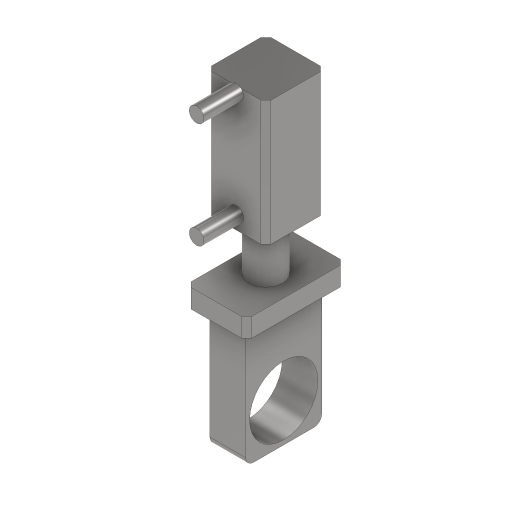
# Autodesk Inventor part: Gatevalve_70_pneumatic
Saved by Autodesk Inventor 2024.2 (Build 282272000, 272)
## iProperties
Created: 2022-11-16
Part Number: Gatevalve_70_pneumatic
Material: Stainless Steel, 440C
Document SubType Name: Modeling
Designer: kuzmin
Density: 7.75 g/cm^3
Appearance: Semi-Polished
Author: kuzmin
Autodesk Inventor part; units mm, degrees
ref_plane "YZ Plane" through (0, 0, 0) normal (1, 0, 0) x (0, 1, 0)
ref_plane "XZ Plane" through (0, 0, 0) normal (0, 1, 0) x (-1, 0, 0)
ref_plane "XY Plane" through (0, 0, 0) normal (0, 0, 1) x (1, 0, 0)
sketch "Sketch1" plane through (0, 0, 0) normal (0, 1, 0) x (-1, 0, 0)
  line L0 (18, 38.5) -> (-18, 38.5)
  line L1 (-18, 38.5) -> (-18, -38.5)
  line L2 (-18, -38.5) -> (18, -38.5)
  line L3 (18, -38.5) -> (18, 38.5)
  line L4 (18, 38.5) -> (-18, -38.5) construction
  point P0 (0, 0)
  point P1 (0, 0)
  dimension "d0" = 77
  dimension "d1" = 36
  constraints: 10 end point, 2 parallel, 1 coincident, 1 horizontal, 1 midpoint, 1 perpendicular
  measures "d0" distance of L2.end L0.start
  measures "d1" distance of L1.end L2.end
extrude "Extrusion1" add sketch "Sketch1" along normal blind 122
sketch "Sketch2" plane through (0, 122, 0) normal (0, 1, 0) x (1, 0, 0)
  line L0 (-30.5, -50) -> (30.5, -50)
  line L1 (30.5, -50) -> (30.5, 50)
  line L2 (30.5, 50) -> (-30.5, 50)
  line L3 (-30.5, 50) -> (-30.5, -50)
  line L4 (-30.5, 50) -> (30.5, -50) construction
  point P0 (0, 0)
  point P1 (0, 0)
  dimension "d4" = 100
  dimension "d5" = 61
  constraints: 10 end point, 2 parallel, 1 coincident, 1 horizontal, 1 midpoint, 1 perpendicular
  measures "d4" distance of L2.end L0.start
  measures "d5" distance of L1.end L2.end
extrude "Extrusion2" add sketch "Sketch2" along normal blind 19
sketch "Sketch3" plane through (0, 141, 0) normal (0, 1, 0) x (1, 0, 0)
  circle A0 centre (0, 0) radius 17
  dimension "d8" = 34
  constraints: 1 centre point, 1 coincident
  measures "d8" diameter of A0
extrude "Extrusion3" add sketch "Sketch3" along normal blind 53
sketch "Sketch4" plane through (0, 194, 0) normal (0, 1, 0) x (1, 0, 0)
  line L0 (-30, -30) -> (30, -30)
  line L1 (30, -30) -> (30, 30)
  line L2 (30, 30) -> (-30, 30)
  line L3 (-30, 30) -> (-30, -30)
  line L4 (-30, 30) -> (30, -30) construction
  point P0 (0, 0)
  point P1 (0, 0)
  dimension "d11" = 60
  constraints: 10 end point, 2 parallel, 2 perpendicular, 1 coincident, 1 horizontal, 1 midpoint
  measures "d11" distance of L2.end L0.start
extrude "Extrusion4" add sketch "Sketch4" along normal blind 126
sketch "Sketch5" plane through (-30, 194, 30) normal (0, 0, 1) x (1, 0, 0)
  circle A0 centre (30, 14) radius 7.5
  line L0 (0, 0) -> (60, 0) projected
  circle A1 centre (30, 121) radius 7.5
  line L1 (0, 126) -> (60, 126) projected
  point P0 (30, -194)
  point P1 (30, 0)
  point P2 (30, 126)
  point P3 (35.5902, 126)
  point P4 (24.4098, 126)
  dimension "d14" = 15
  dimension "d15" = 14
  dimension "d16" = 5
  constraints: 2 centre point, 2 midpoint, 2 vertical alignment, 1 equal radius
  measures "d14" diameter of A0
  measures "d15" distance from line of L0 A0.centre
  measures "d16" distance from line of L1 A1.centre
extrude "Extrusion5" add sketch "Sketch5" along normal blind 40
chamfer "Chamfer1" distance 5 angle 45 4 edges at (30, 257, 30) (30, 257, -30) (-30, 257, -30) (-30, 257, 30)
chamfer "Chamfer2" distance 5 angle 45 4 edges at (30.5, 131.5, -50) (-30.5, 131.5, -50) (-30.5, 131.5, 50) (30.5, 131.5, 50)
fillet "Fillet1" radius 8 2 edges at (0, 0, 38.5) (0, 0, -38.5)
sketch "Sketch6" plane through (18, 122, 38.5) normal (1, 0, 0) x (0, 0, -1)
  circle A0 centre (38.5, -83) radius 34.5
  line L0 (8, -122) -> (69, -122) projected
  point P0 (38.5, -122)
  point P1 (38.5, -122)
  dimension "d26" = 39
  dimension "d27" = 69
  constraints: 1 centre point, 1 midpoint, 1 vertical alignment
  measures "d26" distance from line of L0 A0.centre
  measures "d27" diameter of A0
extrude "Extrusion6" cut sketch "Sketch6" against normal through all
body "Solid1"
